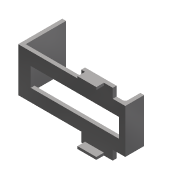
# Autodesk Inventor part: Ultrasonic
Saved by Autodesk Inventor 2018 (Build 220112000, 112)
## iProperties
Created: 2017-11-30
Part Number: Ultrasonic
Material: Stahl, Guss
Document SubType Name: Modeling
Designer: Chris
Density: 7.85 g/cm^3
Appearance: Halbpoliert
Mass: 43.4992 g
Surface Area: 46.0537 cm^2
Volume: 5.5413 cm^3
Author: Chris
Autodesk Inventor part; units mm, degrees
ref_plane "YZ Plane" through (0, 0, 0) normal (1, 0, 0) x (0, 1, 0)
ref_plane "XZ Plane" through (0, 0, 0) normal (0, 1, 0) x (-1, 0, 0)
ref_plane "XY Plane" through (0, 0, 0) normal (0, 0, 1) x (1, 0, 0)
sketch "Skizze1" plane through (0, 0, 0) normal (0, 1, 0) x (-1, 0, 0)
  line L0 (0, 0) -> (25, 0)
  line L1 (25, 50) -> (0, 50)
  line L2 (0, 42.5) -> (-9.9167, 42.5)
  line L3 (-9.9167, 42.5) -> (-9.9167, 7.5)
  line L4 (-9.9167, 7.5) -> (0, 7.5)
  line L5 (65, 32.5) -> (-5, 32.5)
  line L6 (-5, 32.5) -> (-5, 17.5)
  line L7 (-5, 17.5) -> (65, 17.5)
  line L8 (65, 17.5) -> (65, 32.5)
  line L9 (0, 7.5) -> (0, 17.5)
  line L10 (0, 32.5) -> (0, 42.5)
  line L11 (0, 50) -> (0, 32.5)
  line L12 (0, 17.5) -> (0, 0)
  line L13 (25, 42.5) -> (75, 42.5)
  line L14 (75, 42.5) -> (75, 7.5)
  line L15 (75, 7.5) -> (25, 7.5)
  line L16 (25, 0) -> (25, 17.5)
  line L17 (25, 32.5) -> (25, 50)
  dimension "d0" = 50
  dimension "d1" = 25
  dimension "d2" = 7.5
  dimension "d4" = 35
  dimension "d5" = 10
  dimension "d6" = 15
  dimension "d8" = 70
  dimension "d9" = 65
  dimension "d26" = 50
  dimension "d27" = 35
  dimension "d28" = 7.5
  constraints: 36 end point, 10 parallel, 7 perpendicular, 7 point on line, 4 horizontal
  measures "d0" distance of L0.end L1.start
  measures "d1" distance of L1.start L1.end
  measures "d2" distance between parallel lines of L1 L2
  measures "d4" distance of L2.end L3.end
  measures "d5" distance between parallel lines of L2 L5
  measures "d6" distance of L7.end L5.start
  measures "d8" distance of L6.end L7.end
  measures "d9" distance between parallel lines of L10 L8
  measures "d26" distance of L13.start L13.end
  measures "d27" distance between parallel lines of L15 L13
  measures "d28" distance between parallel lines of L1 L13
extrude "Extrusion1" add sketch "Skizze1" along normal blind 3 contours L12 L9 L7 L16 L0 | L4 L3 L2 L10 L5 L6 L7 L9 | L16 L7 L8 L5 L17 L13 L14 L15 | L11 L1 L17 L5 L10
sketch "Skizze2" plane through (0, 0, 42.5) normal (0, 0, 1) x (1, 0, 0)
  line L0 (9.9167, 0) -> (9.9167, 3) projected
  line L1 (9.9167, 3) -> (6.9167, 3)
  line L2 (6.9167, 3) -> (6.9167, 15)
  line L3 (6.9167, 15) -> (9.9167, 15)
  line L4 (9.9167, 15) -> (9.9167, 3)
  point P0 (0, 0)
  dimension "d12" = 3
  dimension "d13" = 12
  constraints: 8 end point, 2 parallel, 1 horizontal, 1 perpendicular
  measures "d12" distance of L2.end L3.end
  measures "d13" distance of L1.end L2.end
extrude "Extrusion2" add sketch "Skizze2" against normal up to surface (35 mm away)
fillet "Rundung1" radius 2 1 edges at (6.9167, 3, 25)
sketch "Skizze3" plane through (0, 0, 0) normal (0, -1, 0) x (1, 0, 0)
  line L0 (-22, 0) -> (-7, 0)
  line L1 (-7, 0) -> (-7, 2)
  line L2 (-7, 2) -> (-22, 2)
  line L3 (-22, 2) -> (-22, 0)
  line L4 (-22, 48) -> (-7, 48)
  line L5 (-7, 48) -> (-7, 50)
  line L6 (-7, 50) -> (-22, 50)
  line L7 (-22, 50) -> (-22, 48)
  line L8 (-25, 50) -> (0, 50) projected
  line L9 (0, 50) -> (0, 42.5) projected
  point P0 (0, 0)
  point P1 (0, 32.5)
  dimension "d17" = 2
  dimension "d18" = 2
  dimension "d19" = 46
  dimension "d20" = 15
  dimension "d21" = 15
  dimension "d22" = 0
  dimension "d23" = 7
  constraints: 16 end point, 4 parallel, 2 horizontal, 2 perpendicular, 1 point on line
  measures "d17" distance between parallel lines of L0 L2
  measures "d18" distance of L6.end L4.start
  measures "d19" distance between parallel lines of L4 L2
  measures "d20" distance of L1.end L2.end
  measures "d21" distance of L5.end L6.end
  measures "d22" distance between parallel lines of L8 L6
  measures "d23" distance between parallel lines of L9 L5
extrude "Extrusion3" add sketch "Skizze3" along normal blind 6
sketch "Skizze4" plane through (-75, 0, 7.5) normal (-1, 0, 0) x (0, 0, 1)
  line L0 (0, 0) -> (0, 35)
  line L1 (0, 35) -> (35, 35)
  line L2 (35, 0) -> (35, 15) projected
  line L3 (35, 35) -> (35, 0)
  line L4 (0, 0) -> (0, 15) projected
  line L5 (35, 0) -> (0, 0)
  point P0 (-7.5, 0)
  dimension "d29" = 35
  constraints: 8 end point, 3 perpendicular, 1 vertical
  measures "d29" distance of L0.start L0.end
extrude "Extrusion4" add sketch "Skizze4" against normal blind 3
fillet "Rundung2" radius 7 1 edges at (-72, 3, 25)
